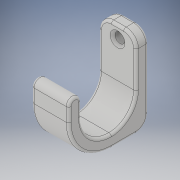
# Autodesk Inventor part: single_hook
Saved by Autodesk Inventor 2019 (Build 230136000, 136)
## iProperties
Created: 2019-02-20
Part Number: single_hook
Material: Generic
Document SubType Name: Modeling
Designer: jmc
Density: 1 g/cm^3
Appearance: Default
Author: jmc
Autodesk Inventor part; units mm, degrees
ref_plane "YZ Plane" through (0, 0, 0) normal (1, 0, 0) x (0, 1, 0)
ref_plane "XZ Plane" through (0, 0, 0) normal (0, 1, 0) x (-1, 0, 0)
ref_plane "XY Plane" through (0, 0, 0) normal (0, 0, 1) x (1, 0, 0)
sketch "Sketch1" plane through (0, 0, 0) normal (0, 0, 1) x (1, 0, 0)
  line L0 (-2.5, 25) -> (2.5, 25)
  line L1 (7.5, 20) -> (7.5, -20)
  line L2 (2.5, -25) -> (-2.5, -25)
  line L3 (-7.5, -20) -> (-7.5, 20)
  line L4 (-7.5, 25) -> (7.5, -25) construction
  line L5 (7.5, 25) -> (-7.5, -25) construction
  arc A0 (-2.5, 25) -> (-7.5, 20) centre (-2.5, 20) ccw
  arc A1 (7.5, 20) -> (2.5, 25) centre (2.5, 20) ccw
  arc A2 (2.5, -25) -> (7.5, -20) centre (2.5, -20) ccw
  arc A3 (-7.5, -20) -> (-2.5, -25) centre (-2.5, -20) ccw
  circle A4 centre (0, 20) radius 1
  point P0 (0, 0)
  dimension "d0" = 15
  dimension "d1" = 50
  dimension "d2" = 5
  dimension "d5" = 2
  constraints: 12 end point, 8 point on circle, 8 point on line, 8 tangent, 5 centre point, 3 equal radius, 2 midpoint, 2 parallel, 1 coincident, 1 horizontal, 1 perpendicular
  measures "d0" distance of L4.end L5.end
  measures "d1" distance of L5.start L4.end
  measures "d2" radius of A0
  measures "d5" diameter of A4
extrude "Extrusion2" add sketch "Sketch1" along normal blind 5
sketch "Sketch3" plane through (0, 0, 5) normal (0, 0, 1) x (1, 0, 0)
  circle A0 centre (0, 20) radius 1 projected
  point P0 (0, 0)
  constraints: 1 coincident
hole "Hole1" at (0, 20, 5) direction (0, 0, -1) diameter 4 end through all countersink diameter 6 countersink angle 90
sketch "Sketch4" plane through (0, 0, 0) normal (1, 0, 0) x (0, 1, 0)
  line L0 (28.9186, 2.2501) -> (-11.8341, 2.2501) construction
  line L1 (20, 0) -> (-20, 0) projected
  line L2 (-20, 5) -> (20, 5) construction
  line L3 (-2.191, 5) -> (-11.8341, 5) construction
  line L4 (-7.253, 15) -> (-7.253, 5)
  arc A0 (7.747, 30) -> (-7.253, 15) centre (7.747, 15) ccw
  line L5 (7.747, 30) -> (15.747, 30)
  point P0 (0, 0)
  point P1 (8.5422, 2.2501)
  dimension "d24" = 10
  dimension "d25" = 8
  constraints: 8 end point, 2 horizontal, 2 point on circle, 2 point on line, 2 tangent, 1 centre point, 1 midpoint, 1 perpendicular
  measures "d24" distance of L4.start L4.end
  measures "d25" distance of L5.start L5.end
sketch "Sketch5" plane through (0, 0, 5) normal (0, 0, 1) x (1, 0, 0)
  line L0 (7.5, 20) -> (7.5, -20) projected
  line L1 (-7.5, -4.5373) -> (7.5, -4.5373)
  line L2 (7.5, -4.5373) -> (7.5, -9.5373)
  line L3 (7.5, -9.5373) -> (-7.5, -9.5373)
  line L4 (-7.5, -9.5373) -> (-7.5, -4.5373)
  line L5 (-7.5, -4.5373) -> (7.5, -9.5373) construction
  line L6 (7.5, -4.5373) -> (-7.5, -9.5373) construction
  point P0 (0, 0)
  point P1 (0, -7.0373)
  dimension "d17" = 15
  dimension "d18" = 5
  constraints: 12 end point, 2 midpoint, 2 parallel, 1 horizontal, 1 perpendicular, 1 point on line
  measures "d17" distance of L1.start L1.end
  measures "d18" distance of L3.end L1.start
sweep "Sweep3" add profiles "Sketch5" path "Sketch4" path curves L4 A0 L5
sketch "Sketch8" plane through (0, 0, 5) normal (0, 0, 1) x (1, 0, 0)
  line L0 (7.5, -9.5373) -> (-7.5, -9.5373) projected
  line L1 (-7.5, -4.5373) -> (7.5, -4.5373) projected
  point P0 (0, 0)
sketch "Sketch9" plane through (7.5, -20, 0) normal (1, 0, 0) x (0, 0, -1)
  line L0 (-5, 10.4627) -> (-15.4627, 10.4627)
  line L1 (-5, 10.4627) -> (-15.4627, 10.4627)
  line L2 (-5, 10.4627) -> (-15.4627, 10.4627)
  line L3 (-5, 10.4627) -> (-5, 0) projected
  line L4 (-5, 10.4627) -> (-5, 0)
  arc A0 (-5, 0) -> (-15.4627, 10.4627) centre (-15.4627, 0) ccw
  point P0 (0, 20)
  dimension "d31" = 10.4627
  dimension "d32" = 10.4627
  constraints: 8 end point, 2 point on circle, 1 centre point, 1 collinear, 1 tangent
  measures "d31" distance of L0.end L0.start
  measures "d32" distance of L0.start L3.end
sweep "Sweep4" add profiles "Sketch9" path "Sketch8" path curves L0
sketch "Sketch10" plane through (-7.5, -20, 0) normal (-1, 0, 0) x (0, 0, 1)
  line L0 (27.2843, 27.747) -> (27.2843, 35.747)
  line L1 (32.2843, 27.747) -> (32.2843, 35.747)
  line L2 (27.2843, 35.747) -> (32.2843, 35.747)
  arc A0 (32.2843, 33.247) -> (27.2843, 33.247) centre (29.7843, 33.247) ccw
  line L3 (27.2843, 33.247) -> (27.2843, 35.747)
  line L4 (32.2843, 35.747) -> (32.2843, 33.247)
  line L5 (27.2843, 35.747) -> (32.2843, 35.747)
  point P0 (0, 20)
  point P1 (29.7843, 35.747)
  constraints: 12 end point, 4 tangent, 3 point on circle, 2 point on line, 1 centre point, 1 collinear, 1 horizontal, 1 midpoint
extrude "Extrusion3" cut sketch "Sketch10" against normal through all
sketch "Sketch11" plane through (-7.5, -4.5373, 5) normal (0, 1, 0) x (1, 0, 0)
  line L0 (0, 0) -> (15, 0) projected
  point P0 (7.5, 5)
sketch "Sketch12" plane through (-7.5, -20, 0) normal (-1, 0, 0) x (0, 0, 1)
  line L0 (5, 40) -> (5, 15.4627) projected
  line L1 (5, 15.4627) -> (15, 15.4627) projected
  line L2 (5, 15.4627) -> (15, 15.4627)
  line L3 (5, 15.4627) -> (5, 25.4627)
  line L4 (5, 15.4627) -> (5, 40) projected
  arc A0 (5, 25.4627) -> (15, 15.4627) centre (15, 25.4627) ccw
  point P0 (0, 20)
  dimension "d37" = 10
  constraints: 4 end point, 2 point on circle, 1 centre point, 1 collinear, 1 point on line, 1 tangent
  measures "d37" distance of L0.end L3.end
sweep "Sweep5" add profiles "Sketch12" path "Sketch11"
sketch "Sketch15" plane through (-7.5, -20, 0) normal (-1, 0, 0) x (0, 0, 1)
  arc A0 (5, 25.4627) -> (15, 15.4627) centre (15, 25.4627) ccw projected
  arc A1 (15, 15.4627) -> (27.2843, 27.747) centre (15, 27.747) ccw projected
  line L0 (15.4627, 10.4627) -> (5, 10.4627)
  arc A2 (0, 15.4627) -> (5, 10.4627) centre (5, 15.4627) ccw
  line L1 (0, 0) -> (0, -5) projected
  line L2 (0, -5) -> (5, -5) projected
  line L3 (5, -5) -> (5, 0) projected
  arc A3 (15.4627, 10.4627) -> (5, 0) centre (15.4627, 0) ccw projected
  line L4 (0, 0) -> (5, 0) projected
  line L5 (0, 0) -> (0, 15.4627)
  point P0 (0, 20)
  dimension "d43" = 5
  constraints: 4 end point, 3 point on circle, 2 tangent, 1 centre point, 1 horizontal
  measures "d43" radius of A2
extrude "Extrusion5" cut sketch "Sketch15" against normal through all
fillet "Fillet1" radius 1 26 edges at (7.5, -0.9393, 23.6863) (7.5, 10.497, 27.2843) (7.5, 15.747, 29.7843) (7.5, 10.497, 32.2843) (7.5, -4.4748, 27.2219) (7.5, -9.5373, 10) (7.5, -8.0728, 1.4645) (7.5, 7.7314, 0) (6.0355, 23.5355, 0) (0, 25, 0) (-6.0355, 23.5355, 0) (-7.5, 7.7314, 0) (-7.5, -8.0728, 1.4645) (-7.5, -9.5373, 10) (-7.5, -4.4748, 27.2219) (-7.5, 10.497, 32.2843) (-7.5, 15.747, 29.7843) (-7.5, 10.497, 27.2843) (-7.5, -0.9393, 23.6863) (-7.5, -1.6084, 7.9289) (-7.5, 12.7314, 5) (-6.0355, 23.5355, 5) (0, 25, 5) (6.0355, 23.5355, 5) (7.5, 12.7314, 5) (7.5, -1.6084, 7.9289)
sketch "Sketch13" plane through (7.5, -20, 0) normal (1, 0, 0) x (0, 0, -1)
  arc A0 (-5, 0) -> (-15.4627, 10.4627) centre (-15.4627, 0) ccw projected
  line L0 (0, 0) -> (0, 9.0751)
  line L1 (0, 0) -> (0, 40) projected
  line L2 (0, -5) -> (0, 0) projected
  arc A1 (-5, 0) -> (0, 0) centre (-2.5, 0) ccw
  line L3 (0, -5) -> (-5, -5) projected
  line L4 (0, -5) -> (-5, -5)
  line L5 (-5, 0) -> (-5, -5) projected
  line L6 (-5, -5) -> (-5, 0)
  point P0 (0, 20)
  constraints: 7 end point, 2 point on circle, 1 centre point, 1 collinear, 1 horizontal, 1 point on line, 1 tangent
equation "\"d31\" = d32"
body "Solid2"
